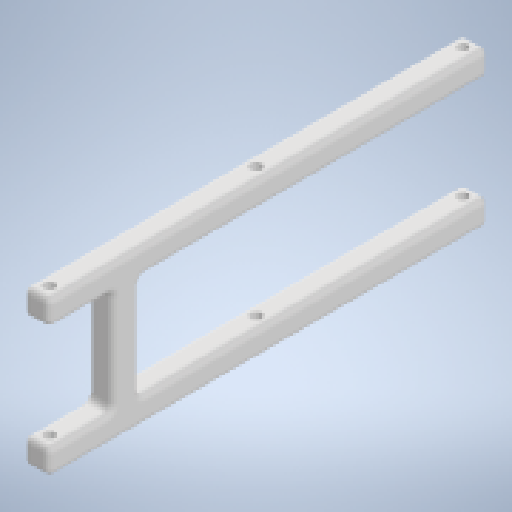
# Autodesk Inventor part: inner swing
Saved by Autodesk Inventor 2023 (Build 270158000, 158)
## iProperties
Created: 2023-01-25
Part Number: inner swing
Material: Generic
Document SubType Name: Modeling
Designer: Gabriel - T3 CAD
Density: 1 g/cm^3
Appearance: Default
Mass: 68.2983 g
Surface Area: 217.239 cm^2
Volume: 68.2983 cm^3
Author: Gabriel - T3 CAD
Autodesk Inventor part; units mm, degrees
ref_plane "YZ Plane" through (0, 0, 0) normal (1, 0, 0) x (0, 1, 0)
ref_plane "XZ Plane" through (0, 0, 0) normal (0, 1, 0) x (-1, 0, 0)
ref_plane "XY Plane" through (0, 0, 0) normal (0, 0, 1) x (1, 0, 0)
sketch "Sketch1" plane through (0, 0, 0) normal (0, 1, 0) x (-1, 0, 0)
  line L0 (0, 0) -> (12.7, 0)
  line L1 (12.7, 0) -> (12.7, 203.2)
  line L2 (12.7, 203.2) -> (0, 203.2)
  line L3 (0, 203.2) -> (0, 0)
  circle A0 centre (6.35, 6.35) radius 2.5797
  circle A1 centre (6.35, 196.85) radius 2.5797
  circle A2 centre (6.35, 101.6) radius 2.5797
  circle A3 centre (6.35, 196.85) radius 6.35
  circle A4 centre (6.35, 6.35) radius 6.35
  point P0 (0, 6.35)
  point P1 (12.7, 6.35)
  point P2 (12.7, 196.85)
  point P3 (0, 196.85)
  point P4 (6.35, 203.2)
  point P5 (6.35, 0)
  dimension "d0" = 12.7
  dimension "d1" = 203.2
  dimension "d2" = 6.35
  dimension "d3" = 6.35
  dimension "d4" = 5.1594
  dimension "d5" = 6.35
  dimension "d6" = 5.1594
  dimension "d7" = 6.35
  dimension "d19" = 5.1594
  dimension "d20" = 6.35
  dimension "d21" = 101.6
  constraints: 8 end point, 5 centre point, 2 coincident, 2 parallel, 1 horizontal, 1 perpendicular
  measures "d0" distance of L2.end L1.end
  measures "d1" distance of L1.end L0.end
  measures "d2" distance from line of L0 A0.centre
  measures "d3" distance from line of L1 A0.centre
  measures "d4" diameter of A0
  measures "d5" distance from line of L1 A1.centre
  measures "d6" diameter of A1
  measures "d7" distance from line of L2 A1.centre
  measures "d19" diameter of A2
  measures "d20" distance from line of L1 A2.centre
  measures "d21" distance from line of L0 A2.centre
extrude "Extrusion1" add sketch "Sketch1" along normal blind 76.2 contours L3 A4 L0 | A4 L1 L0 | A4 | L3 A3 L1 A4 | L3 L2 A3 | A3 | A3 L2 L1 | A0 | A1 | A2
sketch "Sketch3" plane through (0, 0, 203.2) normal (1, 0, 0) x (0, 0, -1)
  line L0 (0, 0) -> (0, 76.2) projected
  line L1 (203.2, 76.2) -> (0, 76.2) projected
  line L2 (0, 0) -> (203.2, 0)
  line L3 (203.2, 0) -> (203.2, 76.2)
  line L4 (203.2, 76.2) -> (0, 76.2)
  line L5 (0, 76.2) -> (0, 0)
  line L6 (203.2, 0) -> (203.2, 76.2) projected
  line L7 (203.2, 63.5) -> (0, 63.5)
  line L8 (0, 63.5) -> (0, 12.7)
  line L9 (0, 12.7) -> (203.2, 12.7)
  line L10 (203.2, 12.7) -> (203.2, 63.5)
  line L11 (0, 63.5) -> (31.75, 63.5)
  line L12 (31.75, 63.5) -> (31.75, 12.7)
  line L13 (31.75, 12.7) -> (0, 12.7)
  line L14 (0, 12.7) -> (0, 63.5)
  line L15 (31.75, 63.5) -> (44.45, 63.5)
  line L16 (44.45, 63.5) -> (44.45, 12.7)
  line L17 (44.45, 12.7) -> (31.75, 12.7)
  line L18 (31.75, 12.7) -> (31.75, 63.5)
  point P0 (44.45, 63.5)
  point P1 (31.75, 63.5)
  point P2 (0, 63.5)
  point P3 (0, 12.7)
  dimension "d27" = 50.8
  dimension "d28" = 12.7
  dimension "d29" = 31.75
  dimension "d30" = 12.7
  constraints: 32 end point, 8 parallel, 4 horizontal, 4 perpendicular, 4 point on line
  measures "d27" distance between parallel lines of L9 L7
  measures "d28" distance between parallel lines of L2 L9
  measures "d29" distance of L12.end L13.end
  measures "d30" distance of L16.end L17.end
extrude "Extrusion3" cut sketch "Sketch3" against normal through all contours L0 L7 L12 L9 | L9 L16 L7 L3
extrude "Extrusion4" cut sketch "Sketch1" along normal through all contours L3 A4 L0 | A4 L1 L0 | L3 L2 A3 | A3 L2 L1 | A0 | A1 | A2
fillet "Fillet2" radius 3.175 28 edges at (-12.7, 38.1, 158.75) (-6.35, 0, 0) (-12.7, 0, 101.6) (-6.35, 0, 203.2) (0, 0, 101.6) (-6.35, 76.2, 203.2) (0, 76.2, 101.6) (-6.35, 76.2, 0) (-12.7, 76.2, 101.6) (-6.35, 63.5, 0) (-12.7, 63.5, 82.55) (0, 63.5, 82.55) (-6.35, 12.7, 0) (0, 12.7, 82.55) (-12.7, 12.7, 82.55) (-6.35, 12.7, 158.75) (0, 38.1, 158.75) (-12.7, 38.1, 171.45) (-6.35, 12.7, 171.45) (-6.35, 63.5, 171.45) (-6.35, 12.7, 203.2) (0, 12.7, 184.15) (-12.7, 12.7, 184.15) (-6.35, 63.5, 203.2) (0, 63.5, 184.15) (-12.7, 63.5, 184.15) (0, 38.1, 171.45) (-6.35, 63.5, 158.75)
equation "\"d21\" = 0.5 * d1"
body "Solid1"
